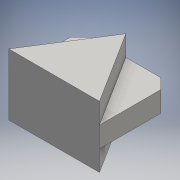
# Autodesk Inventor part: 240503_3Dsketch08
Saved by Autodesk Inventor 2016 (Build 200138000, 138)
## iProperties
Created: 2024-05-03
Part Number: 240503_3Dsketch08
Material: 일반
Document SubType Name: Modeling
Designer: pc
Density: 1 g/cm^3
Appearance: 기본값
Author: pc
Autodesk Inventor part; units mm, degrees
ref_plane "YZ Plane" through (0, 0, 0) normal (1, 0, 0) x (0, 1, 0)
ref_plane "XZ Plane" through (0, 0, 0) normal (0, 1, 0) x (-1, 0, 0)
ref_plane "XY Plane" through (0, 0, 0) normal (0, 0, 1) x (1, 0, 0)
sketch "스케치1" plane through (0, 0, 0) normal (0, 0, 1) x (1, 0, 0)
  line L0 (22.0682, -17.448) -> (-22.0682, -17.448)
  line L1 (-22.0682, -17.448) -> (-22.0682, 17.448)
  line L2 (-22.0682, 17.448) -> (22.0682, 17.448)
  line L3 (22.0682, 17.448) -> (22.0682, -17.448)
  line L4 (22.0682, -17.448) -> (-22.0682, 17.448) construction
  line L5 (-22.0682, -17.448) -> (22.0682, 17.448) construction
  point P0 (0, 0)
  constraints: 12 end point, 2 midpoint, 2 parallel, 1 horizontal, 1 perpendicular
extrude "돌출1" add sketch "스케치1" along normal blind 10
sketch "스케치2" plane through (0, 0, 10) normal (0, 0, 1) x (1, 0, 0)
  line L0 (22.0682, 17.448) -> (-22.0682, 17.448) projected
  line L1 (-22.0682, -17.448) -> (22.0682, -17.448) projected
  line L2 (0, 17.448) -> (22.0682, -17.448)
  line L3 (0, 17.448) -> (-22.0682, -17.448)
  point P0 (0, 0)
  constraints: 4 end point, 1 midpoint
extrude "돌출2" add sketch "스케치2" along normal blind 10
sketch "스케치3" plane through (0, 0, 0) normal (0, 0, -1) x (-1, 0, 0)
  line L0 (0, 17.448) -> (22.0682, 17.448) projected
  line L1 (-22.0682, -17.448) -> (22.0682, -17.448) projected
  line L2 (0, 17.448) -> (-22.0682, -17.448)
  line L3 (0, 17.448) -> (22.0682, -17.448) projected
  line L4 (22.0682, 17.448) -> (22.0682, -17.448) projected
  line L5 (0, 17.448) -> (22.0682, -17.448)
  point P0 (0, 0)
  constraints: 4 end point, 1 collinear
extrude "돌출3" add sketch "스케치3" along normal blind 10 contours L3 L1 L2
chamfer "모따기1" distance 5 angle 45 1 edges at (22.0682, 17.448, 5)
chamfer "모따기2" distance 5 angle 45 1 edges at (-22.0682, 17.448, 5)
